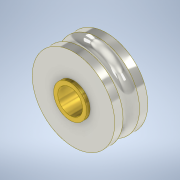
# Autodesk Inventor part: rolik_2
Saved by Autodesk Inventor 2022 (Build 260153000, 153)
## iProperties
Created: 2022-07-30
Part Number: rolik_2
Material: Серебро
Document SubType Name: Modeling
Designer: akapu
Density: 10.49 g/cm^3
Appearance: Серебро
Author: akapu
Autodesk Inventor part; units mm, degrees
ref_plane "YZ Plane" through (0, 0, 0) normal (1, 0, 0) x (0, 1, 0)
ref_plane "XZ Plane" through (0, 0, 0) normal (0, 1, 0) x (-1, 0, 0)
ref_plane "XY Plane" through (0, 0, 0) normal (0, 0, 1) x (1, 0, 0)
sketch "Эскиз6" plane through (0, 0, 0) normal (0, 0, 1) x (1, 0, 0)
  circle A0 centre (0, 0) radius 1.5
  circle A1 centre (0, 0) radius 5
  dimension "d16" = 3
  dimension "d30" = 10
  constraints: 2 centre point, 1 coincident
  measures "d16" diameter of A0
  measures "d30" diameter of A1
extrude "Выдавливание5" add sketch "Эскиз6" along normal blind 4
sketch "Эскиз7" plane through (0, 0, 0) normal (0, 1, 0) x (-1, 0, 0)
  line L0 (0, 0) -> (0, 4)
  line L1 (5, 4) -> (-5, 4) projected
  line L2 (5, 0) -> (5, 4) projected
  line L3 (5, 2) -> (4.5, 2)
  line L4 (5, 2) -> (5, 1)
  line L5 (5, 0) -> (5, 4) projected
  line L6 (5, 1) -> (5, 3)
  line L7 (5, 0) -> (5, 4) projected
  arc A0 (5, 3) -> (5, 1) centre (5.75, 2) ccw
  point P0 (6.5, 6)
  point P1 (6.5, 0)
  point P2 (5, 3)
  point P3 (5, 1)
  dimension "d31" = 0.5
  dimension "d32" = 1
  dimension "d33" = 2
  constraints: 8 end point, 3 point on circle, 2 midpoint, 2 point on line, 1 centre point, 1 horizontal
  measures "d31" distance of L3.start L3.end
  measures "d32" distance of L3.start L4.end
  measures "d33" distance of L4.end L6.end
revolve "Вращение2" cut sketch "Эскиз7" angle 360 about axis through (0, 0, 0) along (0, 0, 1)
fillet "Сопряжение3" [suppressed]
sketch "Эскиз8" plane through (0, 0, 0) normal (0, 0, -1) x (-1, 0, 0)
  circle A0 centre (0, 0) radius 2
  circle A1 centre (0, 0) radius 1.5
  dimension "d25" = 4
  constraints: 2 centre point, 2 coincident
  measures "d25" diameter of A0
extrude "Выдавливание6" add sketch "Эскиз8" along normal blind 0.4 and the other way blind 4.4
